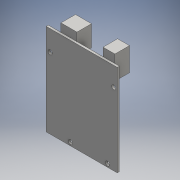
# Autodesk Inventor part: Arduino_Model
Saved by Autodesk Inventor 2016 (Build 200138000, 138)
## iProperties
Created: 2016-06-24
Part Number: Arduino_Model
Material: Generic
Document SubType Name: Modeling
Designer: jorge
Density: 1 g/cm^3
Appearance: Default
Author: jorge
Autodesk Inventor part; units mm, degrees
ref_plane "YZ Plane" through (0, 0, 0) normal (1, 0, 0) x (0, 1, 0)
ref_plane "XZ Plane" through (0, 0, 0) normal (0, 1, 0) x (-1, 0, 0)
ref_plane "XY Plane" through (0, 0, 0) normal (0, 0, 1) x (1, 0, 0)
sketch "Sketch1" plane through (0, 0, 0) normal (0, 1, 0) x (-1, 0, 0)
  line L0 (0, 0) -> (53.3, 0)
  line L1 (53.3, 0) -> (53.3, -68.6)
  line L2 (53.3, -68.6) -> (0, -68.6)
  line L3 (0, -68.6) -> (0, 0)
  dimension "d0" = 68.6
  dimension "d1" = 53.3
  constraints: 8 end point, 2 parallel, 1 horizontal, 1 perpendicular
  measures "d0" distance of L0.end L1.end
  measures "d1" distance of L1.end L2.end
extrude "Extrusion1" add sketch "Sketch1" along normal blind 1.6
sketch "Sketch2" plane through (0, 1.6, 0) normal (0, 1, 0) x (1, 0, 0)
  circle A0 centre (-50.3, 15.3) radius 1.6
  circle A1 centre (-2.5, 14.2) radius 1.6
  circle A2 centre (-7.2, 66.1) radius 1.6
  circle A3 centre (-35.1, 66.1) radius 1.6
  line L0 (-53.3, 0) -> (0, 0) projected
  line L1 (0, 0) -> (0, 68.6) projected
  dimension "d5" = 3.2
  dimension "d6" = 51.9
  dimension "d7" = 50.8
  dimension "d8" = 27.9
  dimension "d9" = 15.2
  dimension "d10" = 4.7
  dimension "d11" = 15.3
  dimension "d12" = 2.5
  constraints: 4 centre point, 3 equal radius, 1 horizontal alignment
  measures "d5" diameter of A3
  measures "d6" vertical distance of A2.centre A1.centre
  measures "d7" vertical distance of A3.centre A0.centre
  measures "d8" distance of A3.centre A2.centre
  measures "d9" horizontal distance of A3.centre A0.centre
  measures "d10" horizontal distance of A2.centre A1.centre
  measures "d11" distance from line of L0 A0.centre
  measures "d12" distance from line of L1 A1.centre
extrude "Extrusion2" cut sketch "Sketch2" against normal through all
sketch "Sketch3" plane through (0, 1.6, 0) normal (0, 1, 0) x (1, 0, 0)
  line L0 (-43.775, 9.525) -> (-31.775, 9.525)
  line L1 (-31.775, 9.525) -> (-31.775, -6.2)
  line L2 (-31.775, -6.2) -> (-43.775, -6.2)
  line L3 (-43.775, -6.2) -> (-43.775, 9.525)
  line L4 (-12.2, 11.43) -> (-3.3, 11.43)
  line L5 (-3.3, 11.43) -> (-3.3, -6.2)
  line L6 (-3.3, -6.2) -> (-12.2, -6.2)
  line L7 (-12.2, -6.2) -> (-12.2, 11.43)
  line L8 (-53.3, 0) -> (0, 0) projected
  line L9 (0, 0) -> (0, 68.6) projected
  line L10 (-53.3, 68.6) -> (-53.3, 0) projected
  dimension "d15" = 12
  dimension "d16" = 6.2
  dimension "d18" = 8.9
  dimension "d19" = 3.3
  dimension "d20" = 9.525
  dimension "d21" = 11.43
  dimension "d22" = 9.525
  constraints: 16 end point, 4 parallel, 2 horizontal, 2 perpendicular, 1 point on line
  measures "d15" distance of L1.end L2.end
  measures "d16" distance between parallel lines of L2 L8
  measures "d18" distance of L5.end L6.end
  measures "d19" distance between parallel lines of L9 L5
  measures "d20" distance between parallel lines of L8 L0
  measures "d21" distance between parallel lines of L8 L4
  measures "d22" distance between parallel lines of L10 L3
extrude "Extrusion3" add sketch "Sketch3" along normal blind 10.9
body "Solid1"
